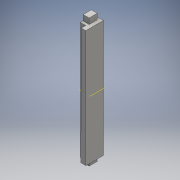
# Autodesk Inventor part: Lower Beam Support
Saved by Autodesk Inventor 2016 (Build 200138000, 138)
## iProperties
Created: 2016-03-08
Part Number: Lower Beam Support
Material: Generic
Document SubType Name: Modeling
Designer: Kenneth Daniel
Density: 1 g/cm^3
Appearance: Default
Mass: 26.8046 g
Surface Area: 91.3783 cm^2
Volume: 26.8046 cm^3
Author: Kenneth Daniel
Autodesk Inventor part; units mm, degrees
ref_plane "YZ Plane" through (0, 0, 0) normal (1, 0, 0) x (0, 1, 0)
ref_plane "XZ Plane" through (0, 0, 0) normal (0, 1, 0) x (-1, 0, 0)
ref_plane "XY Plane" through (0, 0, 0) normal (0, 0, 1) x (1, 0, 0)
sketch "Sketch1" plane through (0, 0, 0) normal (0, 0, 1) x (1, 0, 0)
  line L0 (-5.591, -7.5) -> (-5.591, 7.5)
  line L1 (-5.591, 7.5) -> (5.591, 7.5)
  line L2 (5.591, 7.5) -> (5.591, -7.5)
  line L3 (5.591, -7.5) -> (-5.591, -7.5)
  line L4 (-5.591, -7.5) -> (5.591, 7.5) construction
  line L5 (-5.591, 7.5) -> (5.591, -7.5) construction
  point P0 (0, 0)
  dimension "d0" = 15
  dimension "d1" = 11.182
  constraints: 12 end point, 2 midpoint, 2 parallel, 1 perpendicular, 1 vertical
  measures "d0" distance of L0.start L0.end
  measures "d1" distance of L0.end L1.end
extrude "Extrusion1" add sketch "Sketch1" along normal blind 133
sketch "Sketch2" plane through (0, 0, 133) normal (0, 0, 1) x (1, 0, 0)
  line L0 (-5.591, 7.5) -> (-5.591, -7.5) projected
  line L1 (-5.591, 0) -> (-5.591, -5)
  line L2 (-5.591, -5) -> (1.909, -5)
  line L3 (1.909, -5) -> (1.909, 5)
  line L4 (5.591, 7.5) -> (-5.591, 7.5) projected
  line L5 (1.909, 5) -> (-5.591, 5)
  line L6 (-5.591, 5) -> (-5.591, 0)
  point P0 (0, 0)
  dimension "d4" = 5
  dimension "d5" = 7.5
  dimension "d6" = 10
  dimension "d7" = 7.5
  constraints: 10 end point, 2 perpendicular, 2 point on line, 1 collinear, 1 midpoint
  measures "d4" distance of L1.start L1.end
  measures "d5" distance of L1.end L2.end
  measures "d6" distance of L2.end L3.end
  measures "d7" distance of L3.end L5.end
extrude "Extrusion2" add sketch "Sketch2" along normal blind 6.5
ref_plane "Work Plane1" through (0, 0, 66.5) normal (0, 0, 1) x (1, 0, 0)
mirror "Mirror1" about plane through (0, 0, 66.5) normal (0, 0, 1) of "Extrusion2"
sketch "Sketch3" plane through (-5.591, -7.5, 0) normal (0, -1, 0) x (1, 0, 0)
  line L0 (0, 133) -> (11.182, 133) projected
  line L1 (11.182, 133) -> (6.182, 133)
  line L2 (6.182, 133) -> (5.591, 0)
  line L3 (11.182, 0) -> (0, 0) projected
  line L4 (5.591, 0) -> (11.182, 0)
  line L5 (11.182, 0) -> (11.182, 133) projected
  line L6 (11.182, 0) -> (11.182, 133)
  line L7 (0, 0) -> (0, 133) projected
  dimension "d10" = 5
  constraints: 8 end point, 1 parallel, 1 point on line
  measures "d10" distance of L0.end L1.end
extrude "Extrusion3" add sketch "Sketch3" along normal blind 5 contours L0 L5 L3 L2
sketch "Sketch4" plane through (0, 0, 139.5) normal (0, 0, 1) x (1, 0, 0)
  line L0 (-5.591, 5) -> (-5.591, -5) projected
  line L1 (-5.591, -5) -> (1.909, -5) projected
  line L2 (1.909, -5) -> (1.909, 5) projected
  line L3 (1.909, 5) -> (-5.591, 5) projected
  line L4 (-5.191, -4.6) -> (-5.191, 4.6)
  line L5 (-5.191, 4.6) -> (1.509, 4.6)
  line L6 (1.509, 4.6) -> (1.509, -4.6)
  line L7 (1.509, -4.6) -> (-5.191, -4.6)
  point P0 (0, 0)
  dimension "d13" = 0.4
  constraints: 8 end point, 3 other
  measures "d13" distance between parallel lines of L0 L4
extrude "Extrusion4" cut sketch "Sketch4" against normal up to surface (6.5 mm away)
mirror "Mirror2" about plane through (0, 0, 66.5) normal (0, 0, 1) of "Extrusion4"
ref_plane "Work Plane2" through (0, 0, 66.5) normal (0, 0, 1) x (1, 0, 0)
body "Solid1"
